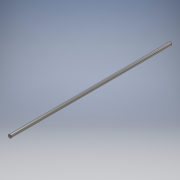
# Autodesk Inventor part: fc17-140
Saved by Autodesk Inventor 2017.1 (Build 211199000, 199)
## iProperties
Category: Miscellaneous
Company: Autodesk Inc.
Created: 2016-12-21
Part Number: fc17-140
Material: Stainless Steel
Document SubType Name: Modeling
Designer: Autodesk Inc.
Density: 8 g/cm^3
Appearance: Semi-Polished
Catalog Web Link: https://us.misumi-ec.com/vona2/detail/110300086920/?HissuCode=SSFHR10-%5B15-600%2F0.1%5D&PNSearch=SSFHR10-500&CategorySpec=00000029631%3A%3A500&KWSearch=SSFHR10-500&Keyword=SSFHR10-500&searchFlow=results2products&Keyword=SSFHR10-500
Vendor: AndyMark Inc
Author: Autodesk Inc.
Title: SSFHR10-500
Keywords: FIRST Choice
Autodesk Inventor part; units mm, degrees
ref_plane "YZ Plane" through (0, 0, 0) normal (1, 0, 0) x (0, 1, 0)
ref_plane "XZ Plane" through (0, 0, 0) normal (0, 1, 0) x (-1, 0, 0)
ref_plane "XY Plane" through (0, 0, 0) normal (0, 0, 1) x (1, 0, 0)
sketch "Sketch1" plane through (0, 0, 0) normal (0, 1, 0) x (-1, 0, 0)
  circle A0 centre (0, 0) radius 5
  dimension "d0" = 10
  constraints: 1 centre point, 1 coincident
  measures "d0" diameter of A0
extrude "Extrusion1" add sketch "Sketch1" against normal blind 500
chamfer "Chamfer1" distance 0.5 angle 45 2 edges at (5, 0, 0) (5, -500, 0)
body "Solid1"
